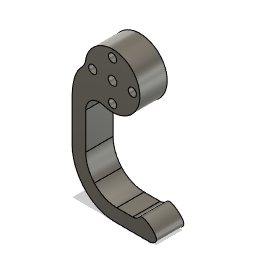
End Effector (Autodesk Fusion 360 archive; units mm, degrees)
design "Handle Lock"
Autodesk Fusion 360 part; units mm, degrees
sketch "Sketch1" plane through (0, 0, 0) normal (0, 0, 1) x (1, 0, 0)
  circle A0 centre (0, 22.5) radius 2.5
  circle A1 centre (0, -22.5) radius 2.5
  arc A2 (0, 25) -> (0, -25) centre (0, 0) ccw
  arc A3 (0, 20) -> (0, -20) centre (0, 0) ccw
  dimension "d1" = 5
  dimension "d2" = 5
  dimension "d3" = 45
  dimension "d8" = 22.5
  constraint vertical A0.centre A1.centre
  constraint vertical A2.centre A1.centre
  constraint coincident A1 A2.end
  constraint coincident A0 A2.start
  constraint coincident A2.centre A3.centre
  constraint vertical A0.centre A2.start
  constraint coincident A1 A3.end
  constraint coincident A0 A3.start
  constraint vertical A0.centre A3.start
  measures "d1" diameter of A1
  measures "d2" diameter of A0
  measures "d3" distance of A0.centre A1.centre
  measures "d8" distance of A2.centre A0.centre
sketch "Sketch2" plane through (0, 0, 0) normal (0, 0, 1) x (1, 0, 0)
  line L0 (-2.2001, -21.9635) -> (14, -21.9635)
  spline S0 degree 5 poles (-0.5432, 24.8315) (-1.4306, 24.8012) (-3.1687, 24.6706) (-5.6653, 24.2644) (-8.7582, 23.2732) (-12.0383, 20.9182) (-13.8982, 17.5787) (-14.6475, 13.8443) (-14.8141, 10.7205) (-14.8141, 9) knots 0 0 0 0 0 0 0.2 0.4 0.6 0.8 1 1 1 1 1 1
  line L1 (-14.8141, 13) -> (-14.8141, 5)
  spline S1 degree 5 poles (14, -21.9635) (14.1337, -21.9186) (14.3908, -21.8256) (14.7461, -21.6764) (15.1586, -21.4579) (15.57, -21.1515) (15.8724, -20.8099) (16.0588, -20.4306) (16.1188, -20.0094) (16.0396, -19.5412) (15.8102, -19.0235) (15.4265, -18.4594) (14.8949, -17.8607) (14.2387, -17.2525) (13.5003, -16.6742) (12.7318, -16.1704) (11.988, -15.7842) (11.3186, -15.5488) (10.7598, -15.4796) (10.328, -15.5669) (10.0079, -15.7637) (9.8137, -15.9552) (9.6872, -16.091) (9.6092, -16.1744) (9.5717, -16.2142) knots 0 0 0 0 0 0 0.05 0.1 0.15 0.2 0.25 0.3 0.35 0.4 0.45 0.5 0.55 0.6 0.65 0.7 0.75 0.8 0.85 0.9 0.95 1 1 1 1 1 1
  spline S2 degree 3 poles (0.2065, 19.8031) (-2.0241, 19.7838) (-4.0258, 19.452) (-5.4795, 18.8912) (-6.3977, 18.537) (-7.0668, 18.1228) (-7.6068, 17.5883) (-8.139, 17.0614) (-8.6149, 16.3967) (-9.0447, 15.0827) (-9.4826, 13.7438) (-9.8141, 11.6994) (-9.8141, 8.8031) knots 0.00097 0.00097 0.00097 0.00097 0.34681 0.34681 0.34681 0.565273 0.565273 0.565273 0.780592 0.780592 0.780592 1 1 1 1
  line L2 (-9.8141, 8.8031) -> (-9.8141, -5.1959)
  line L3 (1.5518, -17.1594) -> (7.3859, -17.1594)
  arc A0 (7.3859, -17.1594) -> (9.5717, -16.2142) centre (7.3859, -14.1594) ccw
  arc A1 (0.2065, 19.8031) -> (-0.5432, 24.8315) centre (0.0014, 22.3426) ccw
  arc A2 (-9.8141, -5.1959) -> (-6.6748, -13.4617) centre (2.6373, -5.1959) ccw
  arc A3 (-14.8141, -5.1959) -> (-2.2001, -21.9635) centre (2.6373, -5.1959) ccw
  line L4 (-14.8141, 9) -> (-14.8141, -5.1959)
  arc A4 (-6.6748, -13.4617) -> (1.5518, -17.1594) centre (1.5518, -6.1594) ccw
  point P0 (16, -20.5)
  point P1 (15, -18)
  point P2 (10.67, -15.5248)
  point P3 (18, -17.1594)
  point P4 (-0.8141, -17.1594)
  dimension "d12" = 3
  dimension "d17" = 8.2
  dimension "d18" = 16.2001
  dimension "d19" = 39.502
  dimension "d22" = 11
  constraint midpoint S0.end L1
  constraint parallel L0 L3
  constraint coincident P3 L3
  constraint tangent S1 A0
  constraint tangent L3 A0
  constraint vertical L2
  constraint tangent L2 A2
  constraint tangent A3 L4
  constraint concentric A2 A3
  constraint coincident P4 L3
  constraint coincident P4 A2
  constraint tangent L3 A4
  constraint tangent A2 A4
  measures "d12" radius of A0
  measures "d17" distance of P4 L3.end
  measures "d18" distance of L0.end L0.start
  measures "d19" distance of L3 A1.centre
  measures "d22" radius of A4
extrude "Extrude2" add sketch "Sketch2" along normal blind 10
fillet "Fillet1" radius 15 1 edges at (-2.2001, -21.9635, 5)
sketch "Sketch3" plane through (0, 0, 0) normal (0, 0, -1) x (-1, 0, 0)
  arc A0 (-0.9387, -21.9635) -> (9.4546, -17.7792) centre (-0.9387, -6.9635) ccw
  arc A1 (9.4546, -17.7792) -> (14.8141, -5.1959) centre (-2.6373, -5.1959) ccw
  line L0 (14.8141, -5.1959) -> (14.8141, 9)
  spline S0 degree 5 poles (0.5432, 24.8315) (1.4306, 24.8012) (3.1687, 24.6706) (5.6653, 24.2644) (8.7582, 23.2732) (12.0383, 20.9182) (13.8982, 17.5787) (14.6475, 13.8443) (14.8141, 10.7205) (14.8141, 9) knots 0 0 0 0 0 0 0.2 0.4 0.6 0.8 1 1 1 1 1 1
  arc A2 (0.5432, 24.8315) -> (-0.2065, 19.8031) centre (-0.0014, 22.3426) ccw
  spline S1 degree 3 poles (-0.2065, 19.8031) (2.0241, 19.7838) (4.0258, 19.452) (5.4795, 18.8912) (6.3977, 18.537) (7.0668, 18.1228) (7.6068, 17.5883) (8.139, 17.0614) (8.6149, 16.3967) (9.0447, 15.0827) (9.4826, 13.7438) (9.8141, 11.6994) (9.8141, 8.8031) knots 0.00097 0.00097 0.00097 0.00097 0.34681 0.34681 0.34681 0.565273 0.565273 0.565273 0.780592 0.780592 0.780592 1 1 1 1
  line L1 (9.8141, 8.8031) -> (9.8141, -5.1959)
  arc A3 (6.6748, -13.4617) -> (9.8141, -5.1959) centre (-2.6373, -5.1959) ccw
  arc A4 (-1.5518, -17.1594) -> (6.6748, -13.4617) centre (-1.5518, -6.1594) ccw
  line L2 (-1.5518, -17.1594) -> (-7.3859, -17.1594)
  arc A5 (-9.5717, -16.2142) -> (-7.3859, -17.1594) centre (-7.3859, -14.1594) ccw
  spline S2 degree 5 poles (-14, -21.9635) (-14.1337, -21.9186) (-14.3908, -21.8256) (-14.7461, -21.6764) (-15.1586, -21.4579) (-15.57, -21.1515) (-15.8724, -20.8099) (-16.0588, -20.4306) (-16.1188, -20.0094) (-16.0396, -19.5412) (-15.8102, -19.0235) (-15.4265, -18.4594) (-14.8949, -17.8607) (-14.2387, -17.2525) (-13.5003, -16.6742) (-12.7318, -16.1704) (-11.988, -15.7842) (-11.3186, -15.5488) (-10.7598, -15.4796) (-10.328, -15.5669) (-10.0079, -15.7637) (-9.8137, -15.9552) (-9.6872, -16.091) (-9.6092, -16.1744) (-9.5717, -16.2142) knots 0 0 0 0 0 0 0.05 0.1 0.15 0.2 0.25 0.3 0.35 0.4 0.45 0.5 0.55 0.6 0.65 0.7 0.75 0.8 0.85 0.9 0.95 1 1 1 1 1 1
  line L3 (-14, -21.9635) -> (-0.9387, -21.9635)
  circle A6 centre (-0.0014, 22.3426) radius 10
  circle A7 centre (-0.0014, 29.5926) radius 1.5
  circle A8 centre (-7.2514, 22.3426) radius 1.5
  circle A9 centre (-0.0014, 15.0926) radius 1.5
  circle A10 centre (7.2486, 22.3426) radius 1.5
  dimension "d24" = 3
  dimension "d25" = 7.25
  dimension "d27" = 360
  dimension "d28" = 20
  constraint concentric A2 A6
  constraint vertical A2.centre A7.centre
  measures "d24" diameter of A7
  measures "d25" distance of A2.centre A7.centre
  measures "d28" diameter of A6
extrude "Extrude3" add sketch "Sketch3" against normal up to surface (10 mm away) contours S0 A2 S1 A6 A10 picked at (4.1281, 27.809)
extrude "Extrude4" cut sketch "Sketch3" against normal blind 10 contours S0 A10 picked at (6.9387, 21.5507)
fillet "Fillet2" radius 5 2 edges at (-9.9966, 22.1413, 5) (-8.2892, 16.751, 5)
sketch "Sketch4" plane through (0, 0, 10) normal (0, 0, 1) x (1, 0, 0)
  spline S0 degree 5 poles (-11.2651, 21.0526) (-11.375, 20.9406) (-12.0633, 20.2097) (-13.2121, 18.6352) (-14.1013, 16.5665) (-14.6475, 13.8443) (-14.8141, 10.7205) (-14.8141, 9) knots 0.562635 0.562635 0.562635 0.562635 0.562635 0.562635 0.6 0.8 1 1 1 1 1 1
  line L0 (-14.8141, 9) -> (-14.8141, -5.1959)
  arc A0 (-14.8141, -5.1959) -> (-9.4546, -17.7792) centre (2.6373, -5.1959) ccw
  arc A1 (-9.4546, -17.7792) -> (0.9387, -21.9635) centre (0.9387, -6.9635) ccw
  line L1 (0.9387, -21.9635) -> (14, -21.9635)
  spline S1 degree 5 poles (14, -21.9635) (14.1337, -21.9186) (14.3908, -21.8256) (14.7461, -21.6764) (15.1586, -21.4579) (15.57, -21.1515) (15.8724, -20.8099) (16.0588, -20.4306) (16.1188, -20.0094) (16.0396, -19.5412) (15.8102, -19.0235) (15.4265, -18.4594) (14.8949, -17.8607) (14.2387, -17.2525) (13.5003, -16.6742) (12.7318, -16.1704) (11.988, -15.7842) (11.3186, -15.5488) (10.7598, -15.4796) (10.328, -15.5669) (10.0079, -15.7637) (9.8137, -15.9552) (9.6872, -16.091) (9.6092, -16.1744) (9.5717, -16.2142) knots 0 0 0 0 0 0 0.05 0.1 0.15 0.2 0.25 0.3 0.35 0.4 0.45 0.5 0.55 0.6 0.65 0.7 0.75 0.8 0.85 0.9 0.95 1 1 1 1 1 1
  arc A2 (7.3859, -17.1594) -> (9.5717, -16.2142) centre (7.3859, -14.1594) ccw
  line L2 (7.3859, -17.1594) -> (1.5518, -17.1594)
  arc A3 (-6.6748, -13.4617) -> (1.5518, -17.1594) centre (1.5518, -6.1594) ccw
  arc A4 (-9.8141, -5.1959) -> (-6.6748, -13.4617) centre (2.6373, -5.1959) ccw
  line L3 (-9.8141, -5.1959) -> (-9.8141, 8.1366)
  arc A5 (-3.209, 12.8719) -> (-9.8141, 8.1366) centre (-4.8141, 8.1366) ccw
  arc A6 (-3.209, 12.8719) -> (-9.8894, 23.8166) centre (0.0014, 22.3426) ccw
  spline S2 degree 3 poles (-11.2651, 21.0526) (-10.898, 21.4269) (-10.5921, 21.8565) (-10.125, 22.7951) (-9.9667, 23.2982) (-9.8894, 23.8166) knots 0 0 0 0 0.157256 0.157256 0.314513 0.314513 0.314513 0.314513
  circle A7 centre (7.2514, 22.3426) radius 1.5
  circle A8 centre (0.0014, 29.5926) radius 1.5
  circle A9 centre (0.0014, 15.0926) radius 1.5
  circle A10 centre (-7.2486, 22.3426) radius 1.5
  circle A11 centre (0.0014, 22.3426) radius 1.6
  dimension "d34" = 3.2
  constraint concentric A6 A11
  measures "d34" diameter of A11
extrude "Extrude5" cut sketch "Sketch4" against normal blind 10 contours A11
equation "d8 = d3 / 2"
equation "d17 = 18.2 mm - 10 mm"
equation "d18 = 26.200067 mm - 10 mm"
equation "d25 = ( 14.5 / 2 ) * 1 mm"
